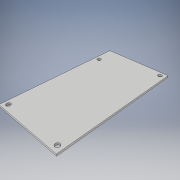
# Autodesk Inventor part: PCB
Saved by Autodesk Inventor 2019 (Build 230136000, 136)
## iProperties
Created: 2019-08-19
Part Number: PCB
Material: Ogólny
Document SubType Name: Modeling
Designer: mikol
Density: 1 g/cm^3
Appearance: Domyślna
Author: mikol
Autodesk Inventor part; units mm, degrees
ref_plane "YZ Plane" through (0, 0, 0) normal (1, 0, 0) x (0, 1, 0)
ref_plane "XZ Plane" through (0, 0, 0) normal (0, 1, 0) x (-1, 0, 0)
ref_plane "XY Plane" through (0, 0, 0) normal (0, 0, 1) x (1, 0, 0)
sketch "Sketch1" plane through (0, 0, 0) normal (0, 1, 0) x (-1, 0, 0)
  circle A0 centre (4.9367, 13.4843) radius 1.75
  line L0 (19.7687, 0) -> (-56.0553, 0) projected
  line L1 (0, -102.5157) -> (0, 37.4843) projected
  circle A1 centre (-41.2233, 13.4843) radius 1.75
  circle A2 centre (-41.2233, -78.5157) radius 1.75
  circle A3 centre (4.9367, -65.5157) radius 1.75
  line L2 (8.9367, 17.4843) -> (-45.2233, 17.4843)
  line L3 (-45.2233, 17.4843) -> (-45.2233, -82.5157)
  line L4 (-45.2233, -82.5157) -> (8.9367, -82.5157)
  line L5 (8.9367, -82.5157) -> (8.9367, 17.4843)
  point P0 (0, 0)
  dimension "d0" = 3.5
  dimension "d3" = 46.16
  dimension "d10" = 92
  dimension "d17" = 79
  dimension "d22" = 4
  dimension "d23" = 4
  dimension "d24" = 4
  dimension "d25" = 4
  dimension "d26" = 4
  constraints: 8 end point, 4 centre point, 2 horizontal, 2 parallel, 2 vertical, 1 perpendicular, 6 other
  measures "d0" diameter of A0
  measures "d3" distance of A0.centre A1.centre
  measures "d10" distance of A1.centre A2.centre
  measures "d17" distance of A0.centre A3.centre
  measures "d22" distance from line of L5 A0.centre
  measures "d23" distance from line of L2 A0.centre
  measures "d24" distance from line of L3 A1.centre
  measures "d25" distance from line of A1.centre L2
  measures "d26" distance from line of L4 A2.centre
extrude "Extrusion1" add sketch "Sketch1" along normal blind 1.6
body "Solid1"
